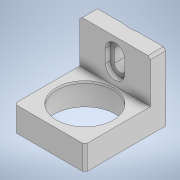
# Autodesk Inventor part: ADAPTER_SM1
Saved by Autodesk Inventor 2020 (Build 240168000, 168)
## iProperties
Created: 2021-02-03
Part Number: ADAPTER_SM1
Material: Generic
Document SubType Name: Modeling
Designer: maria
Density: 1 g/cm^3
Appearance: Default
Mass: 7.93869 g
Surface Area: 46.2203 cm^2
Volume: 7.93869 cm^3
ItemSpecifications: {"_id":"6021a6fc05ba6b0009d58bc4","finish":"543ef1f380da5b0c476373c1","finish_location":null,"material":"5515e170db035c20ce34af9a","process_initialism":null,"quotes":null,"current_quote":null,"quantity_ordered":10,"features":null,"hardware":null,"threading":null,"part_markings":[],"surface_roughness":null,"tolerance":null,"weld_quantity":null,"Notes":"","certifications":[],"part":null,"revision_num":0,"last_history":null,"inspection_requirement_details":{"inspection_requirement":"std","customer_data_sheet":null},"feedback":null}
Author: maria
Autodesk Inventor part; units mm, degrees
ref_plane "YZ Plane" through (0, 0, 0) normal (1, 0, 0) x (0, 1, 0)
ref_plane "XZ Plane" through (0, 0, 0) normal (0, 1, 0) x (-1, 0, 0)
ref_plane "XY Plane" through (0, 0, 0) normal (0, 0, 1) x (1, 0, 0)
sketch "Sketch4" plane through (0, 0, 0) normal (0, 0, 1) x (1, 0, 0)
  line L0 (-14.75, 18) -> (14.7494, 18)
  line L1 (14.7494, 18) -> (14.7494, -10.2)
  line L2 (14.7494, -10.2) -> (-14.75, -10.2)
  line L3 (-14.75, -10.2) -> (-14.75, 18)
  point P0 (0, 0)
  dimension "d24" = 28.2
  dimension "WIDTH" = 29.4994
  dimension "d26" = 14.75
  dimension "d28" = 10.2
  constraints: 8 end point, 2 parallel, 1 horizontal, 1 perpendicular
  measures "d24" distance of L2.end L0.start
  measures "WIDTH" distance of L1.end L2.end
  measures "d26" distance from line of L3 point (0, 0)
  measures "d28" distance from line of L2 point (0, 0)
extrude "Extrusion3" add sketch "Sketch4" against normal blind 6.4
sketch "Sketch5" plane through (0, 0, 0) normal (0, 0, 1) x (1, 0, 0)
  line L0 (-14.75, -10.2) -> (14.7494, -10.2)
  line L1 (14.7494, -10.2) -> (14.7494, 0)
  line L2 (14.7494, 0) -> (-14.75, 0)
  line L3 (-14.75, 0) -> (-14.75, -10.2)
  line L4 (-14.75, 18) -> (-14.75, -10.2) projected
  line L5 (-14.75, -10.2) -> (14.7494, -10.2) projected
  line L6 (14.7494, -10.2) -> (14.7494, 18) projected
  point P0 (0, 0)
  dimension "d31" = 0
  dimension "d32" = 0
  dimension "d33" = 0
  dimension "d34" = 0
  constraints: 8 end point, 2 parallel, 1 horizontal, 1 perpendicular
  measures "d31" distance between parallel lines of L4 L3
  measures "d32" distance between parallel lines of L5 L0
  measures "d33" distance between parallel lines of L6 L1
  measures "d34" distance from line of point (0, 0) L2
extrude "Extrusion4" add sketch "Sketch5" along normal blind 27.4
sketch "Sketch7" plane through (-14.75, -10.2, -6.4) normal (0, -1, 0) x (1, 0, 0)
  circle A0 centre (14.7497, 19.05) radius 12.8397
  line L0 (29.4994, 0) -> (29.4994, 33.8) projected
  line L1 (0, 33.8) -> (29.4994, 33.8) projected
  line L2 (29.4994, 0) -> (0, 0) projected
  dimension "PILOT_HOLE" = 25.6794
  dimension "d201" = 19.05
  dimension "d202" = 14.7497
  constraints: 1 centre point
  measures "PILOT_HOLE" diameter of A0
  measures "d201" distance from line of L2 A0.centre
  measures "d202" distance from line of L0 A0.centre
sketch "Sketch9" plane through (0, 0, -6.4) normal (0, 0, -1) x (-1, 0, 0)
  line L0 (14.75, 18) -> (-14.7494, 18) projected
  line L1 (14.75, 0) -> (-14.7494, 0) projected
  line L2 (0, 6.25) -> (0, 11.75) construction
  line L3 (2.25, 6.25) -> (2.25, 11.75)
  line L4 (-2.25, 11.75) -> (-2.25, 6.25)
  arc A0 (-2.25, 6.25) -> (2.25, 6.25) centre (0, 6.25) ccw
  arc A1 (2.25, 11.75) -> (-2.25, 11.75) centre (0, 11.75) ccw
  line L5 (5.498, 9) -> (4.502, 9) construction
  line L6 (5.498, 10.05) -> (4.502, 10.05)
  line L7 (4.502, 7.95) -> (5.498, 7.95)
  arc A2 (5.498, 7.95) -> (5.498, 10.05) centre (5.498, 9) ccw
  arc A3 (4.502, 10.05) -> (4.502, 7.95) centre (4.502, 9) ccw
  point P0 (0, 0)
  point P1 (-5, 9)
  point P2 (0, 9)
  point P3 (5, 9)
  dimension "d183" = 18
  dimension "d185" = 2.25
  dimension "d186" = 5.5
  dimension "d187" = 0
  dimension "d188" = 9
  dimension "d189" = 1.05
  dimension "d190" = 0.996
  dimension "d191" = 0
  dimension "d192" = 5
  constraints: 16 end point, 8 point on circle, 8 tangent, 4 centre point, 2 midpoint, 2 parallel, 1 horizontal
  measures "d183" distance between parallel lines of L0 L1
  measures "d185" radius of A1
  measures "d186" distance of L2.start L2.end
  measures "d187" horizontal distance of point (0, 0) point (0, 9)
  measures "d188" distance of point (0, 0) point (0, 9)
  measures "d189" radius of A3
  measures "d190" distance of L5.start L5.end
  measures "d191" vertical distance of point (0, 9) point (5, 9)
  measures "d192" distance of point (5, 9) point (0, 9)
extrude "Extrusion6" cut sketch "Sketch9" against normal blind 2.1 contours A2 L7 A3 L6
hole "Hole3" at (5, 9, -6.4) direction (0, 0, 1) diameter 2.1 depth 2.1
extrude "Extrusion7" cut sketch "Sketch7" against normal blind 9.2
sketch "Sketch10" plane through (-0.0003, -1, 12.65) normal (0, -1, 0) x (1, 0, 0)
  circle A0 centre (0, 0) radius 11.85
  circle A1 centre (0, 0) radius 12.8397 projected
  point P0 (0.0003, -12.65)
  point P1 (14.75, 3.9316)
  point P2 (-3.9316, -14.75)
  point P3 (5.6018, -14.2)
  point P4 (-7.6497, 13.2099)
  point P5 (-13.2099, 7.6497)
  point P6 (3.9316, -14.75)
  dimension "d96" = 0
  dimension "d97" = 0
  dimension "d98" = 23.7
  constraints: 1 centre point, 1 other
  measures "d96" distance of point (0, 0) A0.centre
  measures "d97" distance of point (0, 0) A0.centre
  measures "d98" diameter of A0
extrude "Extrusion8" cut sketch "Sketch10" against normal through all contours A0
extrude "Extrusion9" cut sketch "Sketch9" against normal blind 4.386 contours A0 L4 A1 L3
sketch "Sketch11" plane through (0, 0, -2.014) normal (0, 0, -1) x (-1, 0, 0)
  arc A0 (4, 11.75) -> (-4, 11.75) centre (0, 11.75) ccw
  arc A1 (-4, 6.25) -> (4, 6.25) centre (0, 6.25) ccw
  line L0 (-4, 11.75) -> (-4, 6.25)
  line L1 (4, 6.25) -> (4, 11.75)
  point P0 (0, 0)
  point P1 (0, 9)
  dimension "d136" = 8
  dimension "d137" = 8
  dimension "d138" = 0
  dimension "d139" = 5.5
  dimension "d140" = 0
  dimension "d141" = 2.75
  dimension "d142" = 9
  constraints: 4 end point, 4 point on circle, 2 centre point, 1 parallel, 1 tangent, 1 vertical
  measures "d136" diameter of A0
  measures "d137" diameter of A1
  measures "d138" horizontal distance of A1.centre A0.centre
  measures "d139" distance of A0.centre A1.centre
  measures "d140" horizontal distance of A1.centre point (0, 9)
  measures "d141" distance of A0.centre point (0, 9)
  measures "d142" distance of point (0, 0) point (0, 9)
extrude "Extrusion10" cut sketch "Sketch11" against normal through all
chamfer "Chamfer10" distance 1 angle 45 4 edges at (14.7494, -5.1, 27.4) (-14.75, -5.1, 27.4) (14.7494, 18, -3.2) (-14.75, 18, -3.2)
sketch "Sketch13" plane through (-13.75, 18, 0) normal (0, 1, 0) x (1, 0, 0)
  circle A0 centre (13.75, 18.75) radius 12.7
  point P0 (13.75, 0)
  dimension "d196" = 0
  dimension "d197" = 25.4
  dimension "d198" = 18.75
  constraints: 1 centre point
  measures "d196" horizontal distance of point (13.75, 0) A0.centre
  measures "d197" diameter of A0
  measures "d198" distance of point (13.75, 0) A0.centre
extrude "Extrusion11" cut sketch "Sketch13" against normal up to surface (28.2 mm away)
equation "\"d142\" = d131"
equation "\"TOLERANCE\" = 0.05"
equation "\"BEAM_HEIGHT\" = 19.05"
equation "\"d131\" = 9"
body "Solid2"
